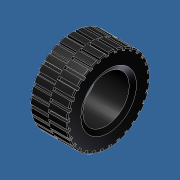
# Autodesk Inventor part: LEGO Brick 3483
Saved by Autodesk Inventor 2011 SP2 (Build 150553200, 553)
## iProperties
Company: Allseas Engineering BV
Created: 2011-11-30
Part Number: LEGO Brick 3483
Cost Center: 0 kg
Material: Steel
Document SubType Name: Modeling
Designer: BvH
Authority: 0 mm^3
Stock Number: =<Filenr>_<Document number>
Density: 7.85 g/cm^3
Mass: 18.9533 g
Surface Area: 18.0068 cm^2
Volume: 2.41443 cm^3
Act. Code: DW000
SaveDate: 2011-07-28
SaveTime: 18:32
FileName: Standard
TotalMass: 0 kg
TotalVolume: 0 mm^3
Subject: =<Title><TITLE 1_2> <TITLE 2_2>
Author: BvH
Autodesk Inventor part; units mm, degrees
ref_plane "YZ Plane" through (0, 0, 0) normal (1, 0, 0) x (0, 1, 0)
ref_plane "XZ Plane" through (0, 0, 0) normal (0, 1, 0) x (-1, 0, 0)
ref_plane "XY Plane" through (0, 0, 0) normal (0, 0, 1) x (1, 0, 0)
sketch "Sketch1" plane through (0, 0, 0) normal (0, 0, 1) x (1, 0, 0)
  line L0 (-4, 12) -> (4, 12)
  line L1 (4, 12) -> (4, 7.5)
  line L2 (4, 7.5) -> (3.4226, 6.5)
  line L3 (3.4226, 6.5) -> (-3.4226, 6.5)
  line L4 (-3.4226, 6.5) -> (-4, 7.5)
  line L5 (-4, 7.5) -> (-4, 12)
  line L6 (0, 5.4) -> (0, 13.1) construction
  line L7 (-5.6, 0) -> (5.6, 0) projected
  point P0 (0, 12)
  point P1 (0, 6.5)
  dimension "d0" = 24
  dimension "d1" = 13
  dimension "d2" = 15
  dimension "d3" = 8
  dimension "d4" = 60
  constraints: 12 end point, 2 horizontal, 2 midpoint, 2 point on line, 2 vertical, 1 parallel
  measures "d0" diameter of L0 L7
  measures "d1" diameter of L3 L7
  measures "d2" diameter of L1.end L7
  measures "d3" distance between parallel lines of L1 L5
  measures "d4" angle of L4 L3
revolve "Revolution1" add sketch "Sketch1" angle 360 about axis through (-10, 0, 0) along (1, 0, 0)
fillet "Fillet1" radius 0.2 2 edges at (4, -12, 0) (-4, -12, 0)
sketch "Sketch2" plane through (0, 0, 0) normal (1, 0, 0) x (0, 1, 0)
  circle A0 centre (0, 0) radius 12 construction
  line L0 (1.2551, 11.9415) -> (0.419, 12)
  line L1 (0.419, 12) -> (0.3981, 11.4)
  line L2 (0.3981, 11.4) -> (1.1924, 11.3445)
  line L3 (1.1924, 11.3445) -> (1.2551, 11.9415)
  line L4 (0, 0) -> (0.8371, 11.9708) construction
  line L5 (-0.419, 12) -> (0.419, 12) construction
  line L6 (0, -14.7) -> (0, 14.7) construction
  point P0 (0, 12)
  dimension "d6" = 0.6
  dimension "d7" = 4
  constraints: 12 end point, 3 point on line, 2 midpoint, 1 equal length, 1 horizontal, 1 parallel, 1 perpendicular, 1 vertical alignment, 2 other
  measures "d6" distance between parallel lines of L2 L0
  measures "d7" angle of L1 L3
extrude "Extrusion1" cut sketch "Sketch2" against normal through all
sketch "Sketch3" plane through (0, 0, 0) normal (1, 0, 0) x (0, 1, 0)
  circle A0 centre (0, 0) radius 12 construction
  line L0 (0, 0) -> (-0.4188, 11.9927) construction
  line L1 (0, 12.0073) -> (0, 11.4069)
  line L2 (0, 11.4069) -> (-0.7957, 11.3792)
  line L3 (-0.7957, 11.3792) -> (-0.8376, 11.9781)
  line L4 (0, 12.0073) -> (-0.8376, 11.9781)
  point P0 (-0.3979, 11.3931)
  dimension "d13" = 0.6
  dimension "d23" = 4
  constraints: 10 end point, 3 point on line, 2 midpoint, 1 perpendicular, 1 vertical, 2 other
  measures "d13" distance between parallel lines of L2 L4
  measures "d23" angle of L1 L3
extrude "Extrusion2" cut sketch "Sketch3" along normal through all
pattern_circular "Circular Pattern2" count 30 over 360 about axis through (-10, 0, 0) along (1, 0, 0) of "Extrusion1", "Extrusion2"
body "Solid1"
